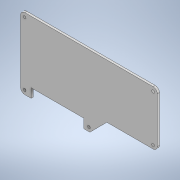
# Autodesk Inventor part: pcb_mockup
Saved by Autodesk Inventor 2021 (Build 250183000, 183)
## iProperties
Created: 2024-09-17
Part Number: pcb_mockup
Material: Generic
Document SubType Name: Modeling
Designer: Toby
Density: 1 g/cm^3
Appearance: Default
Author: Toby
Autodesk Inventor part; units mm, degrees
ref_plane "YZ Plane" through (0, 0, 0) normal (1, 0, 0) x (0, 1, 0)
ref_plane "XZ Plane" through (0, 0, 0) normal (0, 1, 0) x (-1, 0, 0)
ref_plane "XY Plane" through (0, 0, 0) normal (0, 0, 1) x (1, 0, 0)
sketch "Sketch1" plane through (0, 0, 0) normal (0, 0, 1) x (1, 0, 0)
  line L0 (-50, 26) -> (50, 26)
  line L1 (50, 26) -> (50, -26)
  line L2 (50, -26) -> (-50, -26)
  line L3 (-50, -26) -> (-50, 26)
  point P0 (0, 0)
  dimension "d0" = 100
  dimension "d1" = 52
  dimension "d2" = 50
  dimension "d3" = 26
  constraints: 8 end point, 2 parallel, 1 horizontal, 1 perpendicular
  measures "d0" distance of L0.start L0.end
  measures "d1" distance of L2.end L0.start
  measures "d2" distance from line of point (0, 0) L3
  measures "d3" distance from line of point (0, 0) L0
extrude "Extrusion1" add sketch "Sketch1" along normal blind 1.6
sketch "Sketch2" plane through (0, 0, 1.6) normal (0, 0, 1) x (1, 0, 0)
  line L0 (-50, 26) -> (-50, -26) projected
  line L1 (-50, -26) -> (50, -26) projected
  point P0 (0, 0)
  point P1 (-47, -23)
  point P2 (0, -23)
  point P3 (-47, 23)
  point P4 (47, 23)
  point P5 (47, -11)
  dimension "d6" = 3
  dimension "d7" = 3
  dimension "d8" = 50
  dimension "d9" = 3
  dimension "d10" = 97
  dimension "d11" = 15
  dimension "d12" = 3
  dimension "d13" = 49
  dimension "d14" = 97
  dimension "d15" = 49
  measures "d6" distance from line of L0 point (-47, -23)
  measures "d7" distance from line of L1 point (-47, -23)
  measures "d8" distance from line of L0 point (0, -23)
  measures "d9" distance from line of L1 point (0, -23)
  measures "d10" distance from line of L0 point (47, -11)
  measures "d11" distance from line of L1 point (47, -11)
  measures "d12" distance from line of L0 point (-47, 23)
  measures "d13" distance from line of L1 point (-47, 23)
  measures "d14" distance from line of L0 point (47, 23)
  measures "d15" distance from line of L1 point (47, 23)
hole "Hole1" at (-47, -23, 1.6) at (0, -23, 1.6) at (-47, 23, 1.6) at (47, 23, 1.6) at (47, -11, 1.6) direction (0, 0, -1) diameter 2 depth 10 tip angle 118
sketch "Sketch3" plane through (0, 0, 1.6) normal (0, 0, 1) x (1, 0, 0)
  line L0 (-50, -26) -> (50, -26) projected
  line L1 (-42.3, -26) -> (-3.6, -26)
  line L2 (-3.6, -26) -> (-3.6, -19.3)
  line L3 (-3.6, -19.3) -> (-42.3, -19.3)
  line L4 (-42.3, -19.3) -> (-42.3, -26)
  line L5 (50, -26) -> (50, 26) projected
  line L6 (13.1, -26) -> (50, -26)
  line L7 (50, -26) -> (50, -13.5)
  line L8 (50, -13.5) -> (13.1, -13.5)
  line L9 (13.1, -13.5) -> (13.1, -26)
  line L10 (13.1, -13.5) -> (0.7, -26)
  line L11 (0.7, -26) -> (13.1, -26)
  line L12 (-50, 26) -> (-50, -26) projected
  point P0 (0, 0)
  dimension "d23" = 7.7
  dimension "d24" = 6.7
  dimension "d25" = 46.4
  dimension "d26" = 50.7
  dimension "d27" = 63.1
  dimension "d28" = 12.5
  constraints: 20 end point, 4 parallel, 4 point on line, 3 horizontal, 2 perpendicular
  measures "d23" distance between parallel lines of L4 L12
  measures "d24" distance between parallel lines of L0 L3
  measures "d25" distance between parallel lines of L12 L2
  measures "d26" distance from line of L12 L10.end
  measures "d27" distance from line of L12 L8.end
  measures "d28" distance between parallel lines of L0 L8
extrude "Extrusion2" cut sketch "Sketch3" against normal blind 1.6
fillet "Fillet1" radius 3 4 edges at (-50, -26, 0.8) (-50, 26, 0.8) (50, -13.5, 0.8) (50, 26, 0.8)
body "Solid1"
